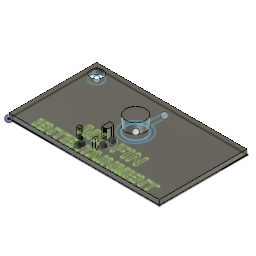
Sotto v2 (Autodesk Fusion 360 design; units mm, degrees)
Autodesk Fusion 360 part; units mm, degrees
sketch "Schizzo1" plane through (0, 0, 0) normal (0, 0, 1) x (1, 0, 0)
  line L0 (0, 0) -> (60, 0)
  line L1 (60, 0) -> (60, 35)
  line L2 (60, 35) -> (0, 35)
  line L3 (0, 35) -> (0, 0)
  circle A0 centre (4, 31) radius 2.5
  line L4 (28.9097, 26.0707) -> (28.9097, 32.0707)
  line L5 (30.9097, 32.0707) -> (30.9097, 26.0707)
  arc A1 (30.9097, 32.0707) -> (28.9097, 32.0707) centre (29.9097, 32.0707) ccw
  circle A2 centre (29.9097, 20.6624) radius 4
  line L6 (19.9916, 9.7411) -> (19.2036, 12.8732)
  line L7 (19.2036, 12.8732) -> (19.2036, 9.4795)
  spline S0 degree 2 poles (19.2036, 9.4795) (19.2036, 9.1979) (19.0778, 9.057) knots 0 0 0 1 1 1
  spline S1 degree 2 poles (19.0778, 9.057) (18.952, 8.9162) (18.7441, 8.9162) knots 0 0 0 1 1 1
  spline S2 degree 2 poles (18.7441, 8.9162) (18.5429, 8.9162) (18.4155, 9.0553) knots 0 0 0 1 1 1
  spline S3 degree 2 poles (18.4155, 9.0553) (18.2881, 9.1945) (18.2881, 9.4795) knots 0 0 0 1 1 1
  line L8 (18.2881, 9.4795) -> (18.2881, 13.3696)
  spline S4 degree 2 poles (18.2881, 13.3696) (18.2881, 13.6915) (18.4557, 13.8038) knots 0 0 0 1 1 1
  spline S5 degree 2 poles (18.4557, 13.8038) (18.6234, 13.9162) (18.9085, 13.9162) knots 0 0 0 1 1 1
  line L9 (18.9085, 13.9162) -> (19.217, 13.9162)
  spline S6 degree 2 poles (19.217, 13.9162) (19.4953, 13.9162) (19.6211, 13.8659) knots 0 0 0 1 1 1
  spline S7 degree 2 poles (19.6211, 13.8659) (19.7468, 13.8156) (19.8072, 13.6848) knots 0 0 0 1 1 1
  spline S8 degree 2 poles (19.8072, 13.6848) (19.8675, 13.554) (19.9447, 13.2589) knots 0 0 0 1 1 1
  line L10 (19.9447, 13.2589) -> (20.659, 10.5661)
  line L11 (20.659, 10.5661) -> (21.3732, 13.2589)
  spline S9 degree 2 poles (21.3732, 13.2589) (21.4504, 13.554) (21.5107, 13.6848) knots 0 0 0 1 1 1
  spline S10 degree 2 poles (21.5107, 13.6848) (21.5711, 13.8156) (21.6968, 13.8659) knots 0 0 0 1 1 1
  spline S11 degree 2 poles (21.6968, 13.8659) (21.8226, 13.9162) (22.1009, 13.9162) knots 0 0 0 1 1 1
  line L12 (22.1009, 13.9162) -> (22.4095, 13.9162)
  spline S12 degree 2 poles (22.4095, 13.9162) (22.6945, 13.9162) (22.8622, 13.8038) knots 0 0 0 1 1 1
  spline S13 degree 2 poles (22.8622, 13.8038) (23.0298, 13.6915) (23.0298, 13.3696) knots 0 0 0 1 1 1
  line L13 (23.0298, 13.3696) -> (23.0298, 9.4795)
  spline S14 degree 2 poles (23.0298, 9.4795) (23.0298, 9.1979) (22.9041, 9.057) knots 0 0 0 1 1 1
  spline S15 degree 2 poles (22.9041, 9.057) (22.7783, 8.9162) (22.5671, 8.9162) knots 0 0 0 1 1 1
  spline S16 degree 2 poles (22.5671, 8.9162) (22.3692, 8.9162) (22.2418, 9.057) knots 0 0 0 1 1 1
  spline S17 degree 2 poles (22.2418, 9.057) (22.1144, 9.1979) (22.1144, 9.4795) knots 0 0 0 1 1 1
  line L14 (22.1144, 9.4795) -> (22.1144, 12.8732)
  line L15 (22.1144, 12.8732) -> (21.3263, 9.7411)
  spline S18 degree 2 poles (21.3263, 9.7411) (21.2492, 9.4359) (21.2005, 9.2934) knots 0 0 0 1 1 1
  spline S19 degree 2 poles (21.2005, 9.2934) (21.1519, 9.1509) (21.0211, 9.0335) knots 0 0 0 1 1 1
  spline S20 degree 2 poles (21.0211, 9.0335) (20.8903, 8.9162) (20.659, 8.9162) knots 0 0 0 1 1 1
  spline S21 degree 2 poles (20.659, 8.9162) (20.4846, 8.9162) (20.3639, 8.9916) knots 0 0 0 1 1 1
  spline S22 degree 2 poles (20.3639, 8.9916) (20.2431, 9.0671) (20.1761, 9.1844) knots 0 0 0 1 1 1
  spline S23 degree 2 poles (20.1761, 9.1844) (20.109, 9.3018) (20.0704, 9.4443) knots 0 0 0 1 1 1
  spline S24 degree 2 poles (20.0704, 9.4443) (20.0319, 9.5869) (19.9916, 9.7411) knots 0 0 0 1 1 1
  line L16 (24.0929, 9.5231) -> (24.0929, 13.3964)
  spline S25 degree 2 poles (24.0929, 13.3964) (24.0929, 13.6982) (24.2304, 13.8491) knots 0 0 0 1 1 1
  spline S26 degree 2 poles (24.2304, 13.8491) (24.3679, 14) (24.5858, 14) knots 0 0 0 1 1 1
  spline S27 degree 2 poles (24.5858, 14) (24.8105, 14) (24.9497, 13.8508) knots 0 0 0 1 1 1
  spline S28 degree 2 poles (24.9497, 13.8508) (25.0889, 13.7015) (25.0889, 13.3964) knots 0 0 0 1 1 1
  line L17 (25.0889, 13.3964) -> (25.0889, 9.5231)
  spline S29 degree 2 poles (25.0889, 9.5231) (25.0889, 9.218) (24.9497, 9.0671) knots 0 0 0 1 1 1
  spline S30 degree 2 poles (24.9497, 9.0671) (24.8105, 8.9162) (24.5858, 8.9162) knots 0 0 0 1 1 1
  spline S31 degree 2 poles (24.5858, 8.9162) (24.3712, 8.9162) (24.2321, 9.0687) knots 0 0 0 1 1 1
  spline S32 degree 2 poles (24.2321, 9.0687) (24.0929, 9.2213) (24.0929, 9.5231) knots 0 0 0 1 1 1
  line L18 (26.8192, 13.9162) -> (28.117, 13.9162)
  spline S33 degree 2 poles (28.117, 13.9162) (28.6234, 13.9162) (28.9856, 13.8223) knots 0 0 0 1 1 1
  spline S34 degree 2 poles (28.9856, 13.8223) (29.3478, 13.7284) (29.6429, 13.4702) knots 0 0 0 1 1 1
  spline S35 degree 2 poles (29.6429, 13.4702) (30.4108, 12.8129) (30.4108, 11.4715) knots 0 0 0 1 1 1
  spline S36 degree 2 poles (30.4108, 11.4715) (30.4108, 11.0288) (30.3337, 10.6633) knots 0 0 0 1 1 1
  spline S37 degree 2 poles (30.3337, 10.6633) (30.2565, 10.2978) (30.0956, 10.0044) knots 0 0 0 1 1 1
  spline S38 degree 2 poles (30.0956, 10.0044) (29.9346, 9.7109) (29.6831, 9.4795) knots 0 0 0 1 1 1
  spline S39 degree 2 poles (29.6831, 9.4795) (29.4852, 9.3018) (29.2505, 9.1945) knots 0 0 0 1 1 1
  spline S40 degree 2 poles (29.2505, 9.1945) (29.0158, 9.0872) (28.7458, 9.0436) knots 0 0 0 1 1 1
  spline S41 degree 2 poles (28.7458, 9.0436) (28.4759, 9) (28.1372, 9) knots 0 0 0 1 1 1
  line L19 (28.1372, 9) -> (26.8394, 9)
  spline S42 degree 2 poles (26.8394, 9) (26.5677, 9) (26.4302, 9.0822) knots 0 0 0 1 1 1
  spline S43 degree 2 poles (26.4302, 9.0822) (26.2928, 9.1643) (26.2508, 9.3135) knots 0 0 0 1 1 1
  spline S44 degree 2 poles (26.2508, 9.3135) (26.2089, 9.4628) (26.2089, 9.7009) knots 0 0 0 1 1 1
  line L20 (26.2089, 9.7009) -> (26.2089, 13.3058)
  spline S45 degree 2 poles (26.2089, 13.3058) (26.2089, 13.6278) (26.3531, 13.772) knots 0 0 0 1 1 1
  spline S46 degree 2 poles (26.3531, 13.772) (26.4973, 13.9162) (26.8192, 13.9162) knots 0 0 0 1 1 1
  line L21 (27.2049, 13.1281) -> (27.2049, 9.7914)
  line L22 (27.2049, 9.7914) -> (27.9594, 9.7914)
  spline S47 degree 2 poles (27.9594, 9.7914) (28.2076, 9.7914) (28.3484, 9.8048) knots 0 0 0 1 1 1
  spline S48 degree 2 poles (28.3484, 9.8048) (28.4893, 9.8182) (28.6402, 9.8719) knots 0 0 0 1 1 1
  spline S49 degree 2 poles (28.6402, 9.8719) (28.7911, 9.9256) (28.9017, 10.0228) knots 0 0 0 1 1 1
  spline S50 degree 2 poles (28.9017, 10.0228) (29.4014, 10.4453) (29.4014, 11.4782) knots 0 0 0 1 1 1
  spline S51 degree 2 poles (29.4014, 11.4782) (29.4014, 12.2059) (29.1818, 12.5681) knots 0 0 0 1 1 1
  spline S52 degree 2 poles (29.1818, 12.5681) (28.9621, 12.9302) (28.6402, 13.0292) knots 0 0 0 1 1 1
  spline S53 degree 2 poles (28.6402, 13.0292) (28.3182, 13.1281) (27.8622, 13.1281) knots 0 0 0 1 1 1
  line L23 (27.8622, 13.1281) -> (27.2049, 13.1281)
  line L24 (34.2237, 13.1482) -> (32.2619, 13.1482)
  line L25 (32.2619, 13.1482) -> (32.2619, 11.8907)
  line L26 (32.2619, 11.8907) -> (33.9017, 11.8907)
  spline S54 degree 2 poles (33.9017, 11.8907) (34.1298, 11.8907) (34.2421, 11.7884) knots 0 0 0 1 1 1
  spline S55 degree 2 poles (34.2421, 11.7884) (34.3545, 11.6861) (34.3545, 11.5151) knots 0 0 0 1 1 1
  spline S56 degree 2 poles (34.3545, 11.5151) (34.3545, 11.3441) (34.2404, 11.2435) knots 0 0 0 1 1 1
  spline S57 degree 2 poles (34.2404, 11.2435) (34.1264, 11.1429) (33.9017, 11.1429) knots 0 0 0 1 1 1
  line L27 (33.9017, 11.1429) -> (32.2619, 11.1429)
  line L28 (32.2619, 11.1429) -> (32.2619, 9.5231)
  spline S58 degree 2 poles (32.2619, 9.5231) (32.2619, 9.2146) (32.1227, 9.0654) knots 0 0 0 1 1 1
  spline S59 degree 2 poles (32.1227, 9.0654) (31.9836, 8.9162) (31.7656, 8.9162) knots 0 0 0 1 1 1
  spline S60 degree 2 poles (31.7656, 8.9162) (31.5443, 8.9162) (31.4051, 9.0671) knots 0 0 0 1 1 1
  spline S61 degree 2 poles (31.4051, 9.0671) (31.2659, 9.218) (31.2659, 9.5231) knots 0 0 0 1 1 1
  line L29 (31.2659, 9.5231) -> (31.2659, 13.3058)
  spline S62 degree 2 poles (31.2659, 13.3058) (31.2659, 13.5205) (31.3296, 13.6563) knots 0 0 0 1 1 1
  spline S63 degree 2 poles (31.3296, 13.6563) (31.3934, 13.7921) (31.5292, 13.8541) knots 0 0 0 1 1 1
  spline S64 degree 2 poles (31.5292, 13.8541) (31.665, 13.9162) (31.8763, 13.9162) knots 0 0 0 1 1 1
  line L30 (31.8763, 13.9162) -> (34.2237, 13.9162)
  spline S65 degree 2 poles (34.2237, 13.9162) (34.4618, 13.9162) (34.5775, 13.8105) knots 0 0 0 1 1 1
  spline S66 degree 2 poles (34.5775, 13.8105) (34.6932, 13.7049) (34.6932, 13.5339) knots 0 0 0 1 1 1
  spline S67 degree 2 poles (34.6932, 13.5339) (34.6932, 13.3595) (34.5775, 13.2539) knots 0 0 0 1 1 1
  spline S68 degree 2 poles (34.5775, 13.2539) (34.4618, 13.1482) (34.2237, 13.1482) knots 0 0 0 1 1 1
  line L31 (35.4745, 9.5231) -> (35.4745, 13.3964)
  spline S69 degree 2 poles (35.4745, 13.3964) (35.4745, 13.6982) (35.612, 13.8491) knots 0 0 0 1 1 1
  spline S70 degree 2 poles (35.612, 13.8491) (35.7495, 14) (35.9675, 14) knots 0 0 0 1 1 1
  spline S71 degree 2 poles (35.9675, 14) (36.1922, 14) (36.3313, 13.8508) knots 0 0 0 1 1 1
  spline S72 degree 2 poles (36.3313, 13.8508) (36.4705, 13.7015) (36.4705, 13.3964) knots 0 0 0 1 1 1
  line L32 (36.4705, 13.3964) -> (36.4705, 9.5231)
  spline S73 degree 2 poles (36.4705, 9.5231) (36.4705, 9.218) (36.3313, 9.0671) knots 0 0 0 1 1 1
  spline S74 degree 2 poles (36.3313, 9.0671) (36.1922, 8.9162) (35.9675, 8.9162) knots 0 0 0 1 1 1
  spline S75 degree 2 poles (35.9675, 8.9162) (35.7529, 8.9162) (35.6137, 9.0687) knots 0 0 0 1 1 1
  spline S76 degree 2 poles (35.6137, 9.0687) (35.4745, 9.2213) (35.4745, 9.5231) knots 0 0 0 1 1 1
  line L33 (38.8816, 13.4031) -> (40.7964, 10.5057)
  line L34 (40.7964, 10.5057) -> (40.7964, 13.4299)
  spline S77 degree 2 poles (40.7964, 13.4299) (40.7964, 13.715) (40.9188, 13.8575) knots 0 0 0 1 1 1
  spline S78 degree 2 poles (40.9188, 13.8575) (41.0412, 14) (41.2492, 14) knots 0 0 0 1 1 1
  spline S79 degree 2 poles (41.2492, 14) (41.4638, 14) (41.5879, 13.8575) knots 0 0 0 1 1 1
  spline S80 degree 2 poles (41.5879, 13.8575) (41.7119, 13.715) (41.7119, 13.4299) knots 0 0 0 1 1 1
  line L35 (41.7119, 13.4299) -> (41.7119, 9.5634)
  spline S81 degree 2 poles (41.7119, 9.5634) (41.7119, 8.9162) (41.1754, 8.9162) knots 0 0 0 1 1 1
  spline S82 degree 2 poles (41.1754, 8.9162) (41.0412, 8.9162) (40.9339, 8.9547) knots 0 0 0 1 1 1
  spline S83 degree 2 poles (40.9339, 8.9547) (40.8266, 8.9933) (40.7327, 9.0771) knots 0 0 0 1 1 1
  spline S84 degree 2 poles (40.7327, 9.0771) (40.6388, 9.161) (40.5583, 9.2733) knots 0 0 0 1 1 1
  spline S85 degree 2 poles (40.5583, 9.2733) (40.4779, 9.3856) (40.3974, 9.503) knots 0 0 0 1 1 1
  line L36 (40.3974, 9.503) -> (38.5295, 12.3669)
  line L37 (38.5295, 12.3669) -> (38.5295, 9.4863)
  spline S86 degree 2 poles (38.5295, 9.4863) (38.5295, 9.2046) (38.3987, 9.0604) knots 0 0 0 1 1 1
  spline S87 degree 2 poles (38.3987, 9.0604) (38.2679, 8.9162) (38.0634, 8.9162) knots 0 0 0 1 1 1
  spline S88 degree 2 poles (38.0634, 8.9162) (37.8521, 8.9162) (37.7247, 9.062) knots 0 0 0 1 1 1
  spline S89 degree 2 poles (37.7247, 9.062) (37.5973, 9.2079) (37.5973, 9.4863) knots 0 0 0 1 1 1
  line L38 (37.5973, 9.4863) -> (37.5973, 13.279)
  spline S90 degree 2 poles (37.5973, 13.279) (37.5973, 13.5205) (37.6509, 13.6579) knots 0 0 0 1 1 1
  spline S91 degree 2 poles (37.6509, 13.6579) (37.7146, 13.8089) (37.8622, 13.9044) knots 0 0 0 1 1 1
  spline S92 degree 2 poles (37.8622, 13.9044) (38.0097, 14) (38.1808, 14) knots 0 0 0 1 1 1
  spline S93 degree 2 poles (38.1808, 14) (38.3149, 14) (38.4105, 13.9564) knots 0 0 0 1 1 1
  spline S94 degree 2 poles (38.4105, 13.9564) (38.506, 13.9128) (38.5781, 13.839) knots 0 0 0 1 1 1
  spline S95 degree 2 poles (38.5781, 13.839) (38.6502, 13.7653) (38.7257, 13.6479) knots 0 0 0 1 1 1
  spline S96 degree 2 poles (38.7257, 13.6479) (38.8011, 13.5305) (38.8816, 13.4031) knots 0 0 0 1 1 1
  line L39 (9.1089, 5.8116) -> (7.3142, 5.7974)
  line L40 (7.3142, 5.7974) -> (7.3218, 4.8316)
  line L41 (7.3218, 4.8316) -> (8.9744, 4.8447)
  spline S97 degree 2 poles (8.9744, 4.8447) (9.1568, 4.8462) (9.2473, 4.7651) knots 0 0 0 1 1 1
  spline S98 degree 2 poles (9.2473, 4.7651) (9.3378, 4.6839) (9.3389, 4.5498) knots 0 0 0 1 1 1
  spline S99 degree 2 poles (9.3389, 4.5498) (9.34, 4.4157) (9.2521, 4.3305) knots 0 0 0 1 1 1
  spline S100 degree 2 poles (9.2521, 4.3305) (9.1642, 4.2453) (8.9791, 4.2438) knots 0 0 0 1 1 1
  line L42 (8.9791, 4.2438) -> (7.3266, 4.2307)
  line L43 (7.3266, 4.2307) -> (7.3355, 3.112)
  line L44 (7.3355, 3.112) -> (9.1919, 3.1267)
  spline S101 degree 2 poles (9.1919, 3.1267) (9.3797, 3.1282) (9.4756, 3.0418) knots 0 0 0 1 1 1
  spline S102 degree 2 poles (9.4756, 3.0418) (9.5715, 2.9554) (9.5727, 2.8105) knots 0 0 0 1 1 1
  spline S103 degree 2 poles (9.5727, 2.8105) (9.5738, 2.671) (9.4793, 2.5831) knots 0 0 0 1 1 1
  spline S104 degree 2 poles (9.4793, 2.5831) (9.3847, 2.4951) (9.1969, 2.4936) knots 0 0 0 1 1 1
  line L45 (9.1969, 2.4936) -> (7.032, 2.4764)
  spline S105 degree 2 poles (7.032, 2.4764) (6.7718, 2.4744) (6.6569, 2.5888) knots 0 0 0 1 1 1
  spline S106 degree 2 poles (6.6569, 2.5888) (6.5419, 2.7033) (6.5399, 2.9608) knots 0 0 0 1 1 1
  line L46 (6.5399, 2.9608) -> (6.5164, 5.9171)
  spline S107 degree 2 poles (6.5164, 5.9171) (6.515, 6.0888) (6.5651, 6.1979) knots 0 0 0 1 1 1
  spline S108 degree 2 poles (6.5651, 6.1979) (6.6153, 6.3069) (6.7235, 6.3574) knots 0 0 0 1 1 1
  spline S109 degree 2 poles (6.7235, 6.3574) (6.8318, 6.4079) (7.0008, 6.4092) knots 0 0 0 1 1 1
  line L47 (7.0008, 6.4092) -> (9.104, 6.4259)
  spline S110 degree 2 poles (9.104, 6.4259) (9.2945, 6.4275) (9.3877, 6.3437) knots 0 0 0 1 1 1
  spline S111 degree 2 poles (9.3877, 6.3437) (9.4809, 6.2599) (9.482, 6.1231) knots 0 0 0 1 1 1
  spline S112 degree 2 poles (9.482, 6.1231) (9.4831, 5.9836) (9.3912, 5.8984) knots 0 0 0 1 1 1
  spline S113 degree 2 poles (9.3912, 5.8984) (9.2993, 5.8131) (9.1089, 5.8116) knots 0 0 0 1 1 1
  line L48 (11.2185, 6.0323) -> (12.7687, 3.7266)
  line L49 (12.7687, 3.7266) -> (12.7502, 6.0659)
  spline S114 degree 2 poles (12.7502, 6.0659) (12.7483, 6.2939) (12.8454, 6.4087) knots 0 0 0 1 1 1
  spline S115 degree 2 poles (12.8454, 6.4087) (12.9424, 6.5235) (13.1087, 6.5248) knots 0 0 0 1 1 1
  spline S116 degree 2 poles (13.1087, 6.5248) (13.2804, 6.5262) (13.3806, 6.413) knots 0 0 0 1 1 1
  spline S117 degree 2 poles (13.3806, 6.413) (13.4807, 6.2997) (13.4825, 6.0717) knots 0 0 0 1 1 1
  line L50 (13.4825, 6.0717) -> (13.5071, 2.9786)
  spline S118 degree 2 poles (13.5071, 2.9786) (13.5112, 2.4608) (13.082, 2.4574) knots 0 0 0 1 1 1
  spline S119 degree 2 poles (13.082, 2.4574) (12.9747, 2.4566) (12.8886, 2.4867) knots 0 0 0 1 1 1
  spline S120 degree 2 poles (12.8886, 2.4867) (12.8025, 2.5169) (12.7269, 2.5834) knots 0 0 0 1 1 1
  spline S121 degree 2 poles (12.7269, 2.5834) (12.6512, 2.6498) (12.5861, 2.7392) knots 0 0 0 1 1 1
  spline S122 degree 2 poles (12.5861, 2.7392) (12.521, 2.8286) (12.4559, 2.9219) knots 0 0 0 1 1 1
  line L51 (12.4559, 2.9219) -> (10.9434, 5.2011)
  line L52 (10.9434, 5.2011) -> (10.9617, 2.8967)
  spline S123 degree 2 poles (10.9617, 2.8967) (10.9635, 2.6713) (10.8598, 2.5551) knots 0 0 0 1 1 1
  spline S124 degree 2 poles (10.8598, 2.5551) (10.7561, 2.4389) (10.5925, 2.4376) knots 0 0 0 1 1 1
  spline S125 degree 2 poles (10.5925, 2.4376) (10.4235, 2.4363) (10.3206, 2.5522) knots 0 0 0 1 1 1
  spline S126 degree 2 poles (10.3206, 2.5522) (10.2177, 2.6681) (10.2159, 2.8907) knots 0 0 0 1 1 1
  line L53 (10.2159, 2.8907) -> (10.1918, 5.9248)
  spline S127 degree 2 poles (10.1918, 5.9248) (10.1903, 6.118) (10.2324, 6.2283) knots 0 0 0 1 1 1
  spline S128 degree 2 poles (10.2324, 6.2283) (10.2824, 6.3495) (10.3998, 6.4268) knots 0 0 0 1 1 1
  spline S129 degree 2 poles (10.3998, 6.4268) (10.5172, 6.5042) (10.654, 6.5053) knots 0 0 0 1 1 1
  spline S130 degree 2 poles (10.654, 6.5053) (10.7614, 6.5062) (10.8381, 6.4719) knots 0 0 0 1 1 1
  spline S131 degree 2 poles (10.8381, 6.4719) (10.9148, 6.4376) (10.973, 6.3791) knots 0 0 0 1 1 1
  spline S132 degree 2 poles (10.973, 6.3791) (11.0311, 6.3205) (11.0922, 6.2271) knots 0 0 0 1 1 1
  spline S133 degree 2 poles (11.0922, 6.2271) (11.1533, 6.1337) (11.2185, 6.0323) knots 0 0 0 1 1 1
  line L54 (16.9104, 5.8307) -> (16.0413, 5.8238)
  line L55 (16.0413, 5.8238) -> (16.064, 2.9667)
  spline S134 degree 2 poles (16.064, 2.9667) (16.0659, 2.7199) (15.9569, 2.5996) knots 0 0 0 1 1 1
  spline S135 degree 2 poles (15.9569, 2.5996) (15.8478, 2.4794) (15.6735, 2.478) knots 0 0 0 1 1 1
  spline S136 degree 2 poles (15.6735, 2.478) (15.4964, 2.4766) (15.3841, 2.5964) knots 0 0 0 1 1 1
  spline S137 degree 2 poles (15.3841, 2.5964) (15.2718, 2.7163) (15.2699, 2.9604) knots 0 0 0 1 1 1
  line L56 (15.2699, 2.9604) -> (15.2472, 5.8174)
  line L57 (15.2472, 5.8174) -> (14.378, 5.8105)
  spline S138 degree 2 poles (14.378, 5.8105) (14.1741, 5.8089) (14.0741, 5.898) knots 0 0 0 1 1 1
  spline S139 degree 2 poles (14.0741, 5.898) (13.9742, 5.9871) (13.973, 6.1346) knots 0 0 0 1 1 1
  spline S140 degree 2 poles (13.973, 6.1346) (13.9718, 6.2875) (14.0744, 6.3769) knots 0 0 0 1 1 1
  spline S141 degree 2 poles (14.0744, 6.3769) (14.1769, 6.4662) (14.3728, 6.4678) knots 0 0 0 1 1 1
  line L58 (14.3728, 6.4678) -> (16.9052, 6.4879)
  spline S142 degree 2 poles (16.9052, 6.4879) (17.1118, 6.4896) (17.2131, 6.3991) knots 0 0 0 1 1 1
  spline S143 degree 2 poles (17.2131, 6.3991) (17.3144, 6.3087) (17.3156, 6.1612) knots 0 0 0 1 1 1
  spline S144 degree 2 poles (17.3156, 6.1612) (17.3168, 6.0136) (17.2156, 5.923) knots 0 0 0 1 1 1
  spline S145 degree 2 poles (17.2156, 5.923) (17.1143, 5.8323) (16.9104, 5.8307) knots 0 0 0 1 1 1
  line L59 (20.3815, 5.9012) -> (18.5868, 5.8869)
  line L60 (18.5868, 5.8869) -> (18.5944, 4.9211)
  line L61 (18.5944, 4.9211) -> (20.247, 4.9343)
  spline S146 degree 2 poles (20.247, 4.9343) (20.4294, 4.9357) (20.5199, 4.8546) knots 0 0 0 1 1 1
  spline S147 degree 2 poles (20.5199, 4.8546) (20.6104, 4.7735) (20.6115, 4.6394) knots 0 0 0 1 1 1
  spline S148 degree 2 poles (20.6115, 4.6394) (20.6126, 4.5052) (20.5247, 4.42) knots 0 0 0 1 1 1
  spline S149 degree 2 poles (20.5247, 4.42) (20.4369, 4.3348) (20.2517, 4.3333) knots 0 0 0 1 1 1
  line L62 (20.2517, 4.3333) -> (18.5992, 4.3202)
  line L63 (18.5992, 4.3202) -> (18.6081, 3.2015)
  line L64 (18.6081, 3.2015) -> (20.4645, 3.2163)
  spline S150 degree 2 poles (20.4645, 3.2163) (20.6523, 3.2178) (20.7482, 3.1313) knots 0 0 0 1 1 1
  spline S151 degree 2 poles (20.7482, 3.1313) (20.8442, 3.0449) (20.8453, 2.9001) knots 0 0 0 1 1 1
  spline S152 degree 2 poles (20.8453, 2.9001) (20.8464, 2.7606) (20.7519, 2.6726) knots 0 0 0 1 1 1
  spline S153 degree 2 poles (20.7519, 2.6726) (20.6573, 2.5847) (20.4695, 2.5832) knots 0 0 0 1 1 1
  line L65 (20.4695, 2.5832) -> (18.3046, 2.566)
  spline S154 degree 2 poles (18.3046, 2.566) (18.0444, 2.5639) (17.9295, 2.6784) knots 0 0 0 1 1 1
  spline S155 degree 2 poles (17.9295, 2.6784) (17.8145, 2.7928) (17.8125, 3.0503) knots 0 0 0 1 1 1
  line L66 (17.8125, 3.0503) -> (17.789, 6.0067)
  spline S156 degree 2 poles (17.789, 6.0067) (17.7877, 6.1783) (17.8378, 6.2874) knots 0 0 0 1 1 1
  spline S157 degree 2 poles (17.8378, 6.2874) (17.8879, 6.3965) (17.9961, 6.4469) knots 0 0 0 1 1 1
  spline S158 degree 2 poles (17.9961, 6.4469) (18.1044, 6.4974) (18.2734, 6.4988) knots 0 0 0 1 1 1
  line L67 (18.2734, 6.4988) -> (20.3766, 6.5155)
  spline S159 degree 2 poles (20.3766, 6.5155) (20.5671, 6.517) (20.6603, 6.4332) knots 0 0 0 1 1 1
  spline S160 degree 2 poles (20.6603, 6.4332) (20.7535, 6.3495) (20.7546, 6.2126) knots 0 0 0 1 1 1
  spline S161 degree 2 poles (20.7546, 6.2126) (20.7557, 6.0731) (20.6638, 5.9879) knots 0 0 0 1 1 1
  spline S162 degree 2 poles (20.6638, 5.9879) (20.572, 5.9027) (20.3815, 5.9012) knots 0 0 0 1 1 1
  line L68 (22.5379, 4.2817) -> (22.2589, 4.2795)
  line L69 (22.2589, 4.2795) -> (22.269, 3.016)
  spline S163 degree 2 poles (22.269, 3.016) (22.271, 2.7665) (22.1619, 2.6476) knots 0 0 0 1 1 1
  spline S164 degree 2 poles (22.1619, 2.6476) (22.0529, 2.5287) (21.8758, 2.5273) knots 0 0 0 1 1 1
  spline S165 degree 2 poles (21.8758, 2.5273) (21.6853, 2.5258) (21.5797, 2.6483) knots 0 0 0 1 1 1
  spline S166 degree 2 poles (21.5797, 2.6483) (21.4741, 2.7709) (21.4722, 3.0097) knots 0 0 0 1 1 1
  line L70 (21.4722, 3.0097) -> (21.4482, 6.0357)
  spline S167 degree 2 poles (21.4482, 6.0357) (21.4461, 6.2933) (21.5606, 6.4095) knots 0 0 0 1 1 1
  spline S168 degree 2 poles (21.5606, 6.4095) (21.675, 6.5258) (21.9326, 6.5278) knots 0 0 0 1 1 1
  line L71 (21.9326, 6.5278) -> (23.2283, 6.5381)
  spline S169 degree 2 poles (23.2283, 6.5381) (23.4966, 6.5403) (23.6872, 6.519) knots 0 0 0 1 1 1
  spline S170 degree 2 poles (23.6872, 6.519) (23.8779, 6.4977) (24.0313, 6.4292) knots 0 0 0 1 1 1
  spline S171 degree 2 poles (24.0313, 6.4292) (24.2171, 6.3528) (24.3604, 6.2091) knots 0 0 0 1 1 1
  spline S172 degree 2 poles (24.3604, 6.2091) (24.5037, 6.0654) (24.579, 5.8741) knots 0 0 0 1 1 1
  spline S173 degree 2 poles (24.579, 5.8741) (24.6543, 5.6829) (24.656, 5.4683) knots 0 0 0 1 1 1
  spline S174 degree 2 poles (24.656, 5.4683) (24.6595, 5.0283) (24.4135, 4.7635) knots 0 0 0 1 1 1
  spline S175 degree 2 poles (24.4135, 4.7635) (24.1674, 4.4986) (23.6639, 4.3846) knots 0 0 0 1 1 1
  spline S176 degree 2 poles (23.6639, 4.3846) (23.8768, 4.2736) (24.0717, 4.0552) knots 0 0 0 1 1 1
  spline S177 degree 2 poles (24.0717, 4.0552) (24.2666, 3.8367) (24.4201, 3.5898) knots 0 0 0 1 1 1
  spline S178 degree 2 poles (24.4201, 3.5898) (24.5736, 3.3428) (24.6597, 3.1436) knots 0 0 0 1 1 1
  spline S179 degree 2 poles (24.6597, 3.1436) (24.7458, 2.9445) (24.7464, 2.8693) knots 0 0 0 1 1 1
  spline S180 degree 2 poles (24.7464, 2.8693) (24.747, 2.7915) (24.698, 2.7147) knots 0 0 0 1 1 1
  spline S181 degree 2 poles (24.698, 2.7147) (24.649, 2.6378) (24.5635, 2.5929) knots 0 0 0 1 1 1
  spline S182 degree 2 poles (24.5635, 2.5929) (24.478, 2.5479) (24.3653, 2.547) knots 0 0 0 1 1 1
  spline S183 degree 2 poles (24.3653, 2.547) (24.2312, 2.546) (24.1395, 2.6083) knots 0 0 0 1 1 1
  spline S184 degree 2 poles (24.1395, 2.6083) (24.0478, 2.6706) (23.9813, 2.7667) knots 0 0 0 1 1 1
  spline S185 degree 2 poles (23.9813, 2.7667) (23.9148, 2.8627) (23.8006, 3.0496) knots 0 0 0 1 1 1
  line L72 (23.8006, 3.0496) -> (23.4772, 3.5783)
  spline S186 degree 2 poles (23.4772, 3.5783) (23.3032, 3.8693) (23.1665, 4.0211) knots 0 0 0 1 1 1
  spline S187 degree 2 poles (23.1665, 4.0211) (23.0298, 4.173) (22.8898, 4.2282) knots 0 0 0 1 1 1
  spline S188 degree 2 poles (22.8898, 4.2282) (22.7499, 4.2834) (22.5379, 4.2817) knots 0 0 0 1 1 1
  line L73 (22.9809, 5.9379) -> (22.2458, 5.9321)
  line L74 (22.2458, 5.9321) -> (22.2544, 4.8509)
  line L75 (22.2544, 4.8509) -> (22.968, 4.8566)
  spline S189 degree 2 poles (22.968, 4.8566) (23.255, 4.8589) (23.4505, 4.9101) knots 0 0 0 1 1 1
  spline S190 degree 2 poles (23.4505, 4.9101) (23.6459, 4.9613) (23.7483, 5.0815) knots 0 0 0 1 1 1
  spline S191 degree 2 poles (23.7483, 5.0815) (23.8506, 5.2017) (23.8489, 5.4109) knots 0 0 0 1 1 1
  spline S192 degree 2 poles (23.8489, 5.4109) (23.8476, 5.5746) (23.7635, 5.6986) knots 0 0 0 1 1 1
  spline S193 degree 2 poles (23.7635, 5.6986) (23.6793, 5.8227) (23.5313, 5.8833) knots 0 0 0 1 1 1
  spline S194 degree 2 poles (23.5313, 5.8833) (23.3913, 5.9412) (22.9809, 5.9379) knots 0 0 0 1 1 1
  line L76 (27.6868, 5.9163) -> (26.8176, 5.9094)
  line L77 (26.8176, 5.9094) -> (26.8403, 3.0523)
  spline S195 degree 2 poles (26.8403, 3.0523) (26.8422, 2.8055) (26.7332, 2.6852) knots 0 0 0 1 1 1
  spline S196 degree 2 poles (26.7332, 2.6852) (26.6241, 2.565) (26.4498, 2.5636) knots 0 0 0 1 1 1
  spline S197 degree 2 poles (26.4498, 2.5636) (26.2727, 2.5622) (26.1604, 2.682) knots 0 0 0 1 1 1
  spline S198 degree 2 poles (26.1604, 2.682) (26.0481, 2.8019) (26.0462, 3.046) knots 0 0 0 1 1 1
  line L78 (26.0462, 3.046) -> (26.0235, 5.903)
  line L79 (26.0235, 5.903) -> (25.1543, 5.8961)
  spline S199 degree 2 poles (25.1543, 5.8961) (24.9504, 5.8945) (24.8505, 5.9836) knots 0 0 0 1 1 1
  spline S200 degree 2 poles (24.8505, 5.9836) (24.7505, 6.0727) (24.7493, 6.2202) knots 0 0 0 1 1 1
  spline S201 degree 2 poles (24.7493, 6.2202) (24.7481, 6.3731) (24.8507, 6.4625) knots 0 0 0 1 1 1
  spline S202 degree 2 poles (24.8507, 6.4625) (24.9533, 6.5518) (25.1491, 6.5534) knots 0 0 0 1 1 1
  line L80 (25.1491, 6.5534) -> (27.6815, 6.5735)
  spline S203 degree 2 poles (27.6815, 6.5735) (27.8881, 6.5752) (27.9894, 6.4847) knots 0 0 0 1 1 1
  spline S204 degree 2 poles (27.9894, 6.4847) (28.0908, 6.3943) (28.0919, 6.2468) knots 0 0 0 1 1 1
  spline S205 degree 2 poles (28.0919, 6.2468) (28.0931, 6.0992) (27.9919, 6.0086) knots 0 0 0 1 1 1
  spline S206 degree 2 poles (27.9919, 6.0086) (27.8906, 5.9179) (27.6868, 5.9163) knots 0 0 0 1 1 1
  line L81 (30.7594, 3.1103) -> (30.5677, 3.6024)
  line L82 (30.5677, 3.6024) -> (28.9689, 3.5897)
  line L83 (28.9689, 3.5897) -> (28.7851, 3.0839)
  spline S207 degree 2 poles (28.7851, 3.0839) (28.6774, 2.7879) (28.6005, 2.684) knots 0 0 0 1 1 1
  spline S208 degree 2 poles (28.6005, 2.684) (28.5235, 2.5801) (28.3464, 2.5787) knots 0 0 0 1 1 1
  spline S209 degree 2 poles (28.3464, 2.5787) (28.1962, 2.5775) (28.08, 2.6866) knots 0 0 0 1 1 1
  spline S210 degree 2 poles (28.08, 2.6866) (27.9637, 2.7956) (27.9626, 2.9351) knots 0 0 0 1 1 1
  spline S211 degree 2 poles (27.9626, 2.9351) (27.962, 3.0156) (27.9881, 3.1017) knots 0 0 0 1 1 1
  spline S212 degree 2 poles (27.9881, 3.1017) (28.0143, 3.1877) (28.0748, 3.3411) knots 0 0 0 1 1 1
  line L84 (28.0748, 3.3411) -> (29.0605, 5.903)
  spline S213 degree 2 poles (29.0605, 5.903) (29.1025, 6.0134) (29.1617, 6.1681) knots 0 0 0 1 1 1
  spline S214 degree 2 poles (29.1617, 6.1681) (29.2208, 6.3228) (29.2884, 6.4253) knots 0 0 0 1 1 1
  spline S215 degree 2 poles (29.2884, 6.4253) (29.356, 6.5278) (29.4668, 6.5917) knots 0 0 0 1 1 1
  spline S216 degree 2 poles (29.4668, 6.5917) (29.5777, 6.6557) (29.7413, 6.657) knots 0 0 0 1 1 1
  spline S217 degree 2 poles (29.7413, 6.657) (29.9076, 6.6583) (30.0195, 6.5961) knots 0 0 0 1 1 1
  spline S218 degree 2 poles (30.0195, 6.5961) (30.1313, 6.534) (30.2005, 6.4352) knots 0 0 0 1 1 1
  spline S219 degree 2 poles (30.2005, 6.4352) (30.2697, 6.3365) (30.3175, 6.2229) knots 0 0 0 1 1 1
  spline S220 degree 2 poles (30.3175, 6.2229) (30.3654, 6.1092) (30.4393, 5.9193) knots 0 0 0 1 1 1
  line L85 (30.4393, 5.9193) -> (31.487, 3.3897)
  spline S221 degree 2 poles (31.487, 3.3897) (31.61, 3.1009) (31.611, 2.9695) knots 0 0 0 1 1 1
  spline S222 degree 2 poles (31.611, 2.9695) (31.6121, 2.8327) (31.499, 2.7177) knots 0 0 0 1 1 1
  spline S223 degree 2 poles (31.499, 2.7177) (31.3859, 2.6028) (31.2249, 2.6015) knots 0 0 0 1 1 1
  spline S224 degree 2 poles (31.2249, 2.6015) (31.131, 2.6008) (31.0637, 2.6338) knots 0 0 0 1 1 1
  spline S225 degree 2 poles (31.0637, 2.6338) (30.9964, 2.6668) (30.9503, 2.7241) knots 0 0 0 1 1 1
  spline S226 degree 2 poles (30.9503, 2.7241) (30.9043, 2.7814) (30.851, 2.9004) knots 0 0 0 1 1 1
  spline S227 degree 2 poles (30.851, 2.9004) (30.7977, 3.0194) (30.7594, 3.1103) knots 0 0 0 1 1 1
  line L86 (29.1734, 4.1896) -> (30.3484, 4.1989)
  line L87 (30.3484, 4.1989) -> (29.7426, 5.8172)
  line L88 (29.7426, 5.8172) -> (29.1734, 4.1896)
  line L89 (32.2271, 3.0951) -> (32.2025, 6.1936)
  spline S228 degree 2 poles (32.2025, 6.1936) (32.2006, 6.435) (32.3096, 6.5566) knots 0 0 0 1 1 1
  spline S229 degree 2 poles (32.3096, 6.5566) (32.4186, 6.6782) (32.593, 6.6796) knots 0 0 0 1 1 1
  spline S230 degree 2 poles (32.593, 6.6796) (32.7727, 6.681) (32.885, 6.5625) knots 0 0 0 1 1 1
  spline S231 degree 2 poles (32.885, 6.5625) (32.9973, 6.444) (32.9992, 6.1999) knots 0 0 0 1 1 1
  line L90 (32.9992, 6.1999) -> (33.0238, 3.1014)
  spline S232 degree 2 poles (33.0238, 3.1014) (33.0258, 2.8573) (32.9154, 2.7357) knots 0 0 0 1 1 1
  spline S233 degree 2 poles (32.9154, 2.7357) (32.805, 2.6141) (32.6253, 2.6127) knots 0 0 0 1 1 1
  spline S234 degree 2 poles (32.6253, 2.6127) (32.4536, 2.6113) (32.3413, 2.7325) knots 0 0 0 1 1 1
  spline S235 degree 2 poles (32.3413, 2.7325) (32.229, 2.8537) (32.2271, 3.0951) knots 0 0 0 1 1 1
  line L91 (34.928, 6.2206) -> (36.4783, 3.9149)
  line L92 (36.4783, 3.9149) -> (36.4597, 6.2542)
  spline S236 degree 2 poles (36.4597, 6.2542) (36.4579, 6.4823) (36.5549, 6.5971) knots 0 0 0 1 1 1
  spline S237 degree 2 poles (36.5549, 6.5971) (36.6519, 6.7118) (36.8182, 6.7132) knots 0 0 0 1 1 1
  spline S238 degree 2 poles (36.8182, 6.7132) (36.9899, 6.7145) (37.0901, 6.6013) knots 0 0 0 1 1 1
  spline S239 degree 2 poles (37.0901, 6.6013) (37.1902, 6.4881) (37.192, 6.2601) knots 0 0 0 1 1 1
  line L93 (37.192, 6.2601) -> (37.2166, 3.1669)
  spline S240 degree 2 poles (37.2166, 3.1669) (37.2207, 2.6492) (36.7915, 2.6458) knots 0 0 0 1 1 1
  spline S241 degree 2 poles (36.7915, 2.6458) (36.6842, 2.6449) (36.5981, 2.6751) knots 0 0 0 1 1 1
  spline S242 degree 2 poles (36.5981, 2.6751) (36.512, 2.7052) (36.4364, 2.7717) knots 0 0 0 1 1 1
  spline S243 degree 2 poles (36.4364, 2.7717) (36.3607, 2.8382) (36.2956, 2.9275) knots 0 0 0 1 1 1
  spline S244 degree 2 poles (36.2956, 2.9275) (36.2305, 3.0169) (36.1654, 3.1103) knots 0 0 0 1 1 1
  line L94 (36.1654, 3.1103) -> (34.6529, 5.3894)
  line L95 (34.6529, 5.3894) -> (34.6712, 3.085)
  spline S245 degree 2 poles (34.6712, 3.085) (34.673, 2.8597) (34.5693, 2.7435) knots 0 0 0 1 1 1
  spline S246 degree 2 poles (34.5693, 2.7435) (34.4656, 2.6273) (34.302, 2.626) knots 0 0 0 1 1 1
  spline S247 degree 2 poles (34.302, 2.626) (34.133, 2.6246) (34.0301, 2.7405) knots 0 0 0 1 1 1
  spline S248 degree 2 poles (34.0301, 2.7405) (33.9272, 2.8564) (33.9255, 3.0791) knots 0 0 0 1 1 1
  line L96 (33.9255, 3.0791) -> (33.9014, 6.1132)
  spline S249 degree 2 poles (33.9014, 6.1132) (33.8998, 6.3063) (33.9419, 6.4167) knots 0 0 0 1 1 1
  spline S250 degree 2 poles (33.9419, 6.4167) (33.9919, 6.5378) (34.1093, 6.6152) knots 0 0 0 1 1 1
  spline S251 degree 2 poles (34.1093, 6.6152) (34.2267, 6.6926) (34.3636, 6.6937) knots 0 0 0 1 1 1
  spline S252 degree 2 poles (34.3636, 6.6937) (34.4709, 6.6945) (34.5476, 6.6603) knots 0 0 0 1 1 1
  spline S253 degree 2 poles (34.5476, 6.6603) (34.6243, 6.626) (34.6825, 6.5674) knots 0 0 0 1 1 1
  spline S254 degree 2 poles (34.6825, 6.5674) (34.7406, 6.5089) (34.8017, 6.4155) knots 0 0 0 1 1 1
  spline S255 degree 2 poles (34.8017, 6.4155) (34.8628, 6.322) (34.928, 6.2206) knots 0 0 0 1 1 1
  line L97 (39.4153, 3.3266) -> (38.7649, 5.8272)
  line L98 (38.7649, 5.8272) -> (38.7865, 3.1123)
  spline S256 degree 2 poles (38.7865, 3.1123) (38.7883, 2.887) (38.6886, 2.7735) knots 0 0 0 1 1 1
  spline S257 degree 2 poles (38.6886, 2.7735) (38.5889, 2.66) (38.4226, 2.6587) knots 0 0 0 1 1 1
  spline S258 degree 2 poles (38.4226, 2.6587) (38.2616, 2.6574) (38.1588, 2.768) knots 0 0 0 1 1 1
  spline S259 degree 2 poles (38.1588, 2.768) (38.056, 2.8785) (38.0541, 3.1065) knots 0 0 0 1 1 1
  line L99 (38.0541, 3.1065) -> (38.0294, 6.2184)
  spline S260 degree 2 poles (38.0294, 6.2184) (38.0274, 6.476) (38.1608, 6.5669) knots 0 0 0 1 1 1
  spline S261 degree 2 poles (38.1608, 6.5669) (38.2942, 6.6578) (38.5222, 6.6596) knots 0 0 0 1 1 1
  line L100 (38.5222, 6.6596) -> (38.769, 6.6616)
  spline S262 degree 2 poles (38.769, 6.6616) (38.9917, 6.6634) (39.0926, 6.6239) knots 0 0 0 1 1 1
  spline S263 degree 2 poles (39.0926, 6.6239) (39.1936, 6.5845) (39.2427, 6.4802) knots 0 0 0 1 1 1
  spline S264 degree 2 poles (39.2427, 6.4802) (39.2918, 6.376) (39.3554, 6.1404) knots 0 0 0 1 1 1
  line L101 (39.3554, 6.1404) -> (39.9439, 3.9908)
  line L102 (39.9439, 3.9908) -> (40.4982, 6.1495)
  spline S265 degree 2 poles (40.4982, 6.1495) (40.558, 6.3861) (40.6055, 6.4911) knots 0 0 0 1 1 1
  spline S266 degree 2 poles (40.6055, 6.4911) (40.6529, 6.5961) (40.7532, 6.6371) knots 0 0 0 1 1 1
  spline S267 degree 2 poles (40.7532, 6.6371) (40.8535, 6.6782) (41.0762, 6.6799) knots 0 0 0 1 1 1
  line L103 (41.0762, 6.6799) -> (41.323, 6.6819)
  spline S268 degree 2 poles (41.323, 6.6819) (41.551, 6.6837) (41.6858, 6.5949) knots 0 0 0 1 1 1
  spline S269 degree 2 poles (41.6858, 6.5949) (41.8207, 6.5061) (41.8227, 6.2485) knots 0 0 0 1 1 1
  line L104 (41.8227, 6.2485) -> (41.8475, 3.1366)
  spline S270 degree 2 poles (41.8475, 3.1366) (41.8492, 2.9113) (41.7495, 2.7978) knots 0 0 0 1 1 1
  spline S271 degree 2 poles (41.7495, 2.7978) (41.6498, 2.6844) (41.4808, 2.683) knots 0 0 0 1 1 1
  spline S272 degree 2 poles (41.4808, 2.683) (41.3225, 2.6818) (41.2197, 2.7936) knots 0 0 0 1 1 1
  spline S273 degree 2 poles (41.2197, 2.7936) (41.1169, 2.9055) (41.1151, 3.1308) knots 0 0 0 1 1 1
  line L105 (41.1151, 3.1308) -> (41.0935, 5.8457)
  line L106 (41.0935, 5.8457) -> (40.483, 3.3351)
  spline S274 degree 2 poles (40.483, 3.3351) (40.4232, 3.0905) (40.3852, 2.9761) knots 0 0 0 1 1 1
  spline S275 degree 2 poles (40.3852, 2.9761) (40.3472, 2.8618) (40.2434, 2.7671) knots 0 0 0 1 1 1
  spline S276 degree 2 poles (40.2434, 2.7671) (40.1395, 2.6724) (39.9544, 2.6709) knots 0 0 0 1 1 1
  spline S277 degree 2 poles (39.9544, 2.6709) (39.8149, 2.6698) (39.7178, 2.7294) knots 0 0 0 1 1 1
  spline S278 degree 2 poles (39.7178, 2.7294) (39.6208, 2.789) (39.5664, 2.8824) knots 0 0 0 1 1 1
  spline S279 degree 2 poles (39.5664, 2.8824) (39.512, 2.9759) (39.4802, 3.0897) knots 0 0 0 1 1 1
  spline S280 degree 2 poles (39.4802, 3.0897) (39.4485, 3.2034) (39.4153, 3.3266) knots 0 0 0 1 1 1
  line L107 (45.2338, 6.0986) -> (43.4391, 6.0843)
  line L108 (43.4391, 6.0843) -> (43.4468, 5.1186)
  line L109 (43.4468, 5.1186) -> (45.0993, 5.1317)
  spline S281 degree 2 poles (45.0993, 5.1317) (45.2817, 5.1331) (45.3723, 5.052) knots 0 0 0 1 1 1
  spline S282 degree 2 poles (45.3723, 5.052) (45.4628, 4.9709) (45.4638, 4.8368) knots 0 0 0 1 1 1
  spline S283 degree 2 poles (45.4638, 4.8368) (45.4649, 4.7027) (45.377, 4.6174) knots 0 0 0 1 1 1
  spline S284 degree 2 poles (45.377, 4.6174) (45.2892, 4.5322) (45.1041, 4.5308) knots 0 0 0 1 1 1
  line L110 (45.1041, 4.5308) -> (43.4516, 4.5176)
  line L111 (43.4516, 4.5176) -> (43.4604, 3.399)
  line L112 (43.4604, 3.399) -> (45.3169, 3.4137)
  spline S285 degree 2 poles (45.3169, 3.4137) (45.5046, 3.4152) (45.6006, 3.3288) knots 0 0 0 1 1 1
  spline S286 degree 2 poles (45.6006, 3.3288) (45.6965, 3.2423) (45.6976, 3.0975) knots 0 0 0 1 1 1
  spline S287 degree 2 poles (45.6976, 3.0975) (45.6988, 2.958) (45.6042, 2.87) knots 0 0 0 1 1 1
  spline S288 degree 2 poles (45.6042, 2.87) (45.5097, 2.7821) (45.3219, 2.7806) knots 0 0 0 1 1 1
  line L113 (45.3219, 2.7806) -> (43.157, 2.7634)
  spline S289 degree 2 poles (43.157, 2.7634) (42.8967, 2.7613) (42.7818, 2.8758) knots 0 0 0 1 1 1
  spline S290 degree 2 poles (42.7818, 2.8758) (42.6669, 2.9902) (42.6648, 3.2478) knots 0 0 0 1 1 1
  line L114 (42.6648, 3.2478) -> (42.6414, 6.2041)
  spline S291 degree 2 poles (42.6414, 6.2041) (42.64, 6.3758) (42.6901, 6.4848) knots 0 0 0 1 1 1
  spline S292 degree 2 poles (42.6901, 6.4848) (42.7402, 6.5939) (42.8485, 6.6444) knots 0 0 0 1 1 1
  spline S293 degree 2 poles (42.8485, 6.6444) (42.9567, 6.6949) (43.1257, 6.6962) knots 0 0 0 1 1 1
  line L115 (43.1257, 6.6962) -> (45.2289, 6.7129)
  spline S294 degree 2 poles (45.2289, 6.7129) (45.4194, 6.7144) (45.5126, 6.6307) knots 0 0 0 1 1 1
  spline S295 degree 2 poles (45.5126, 6.6307) (45.6059, 6.5469) (45.6069, 6.4101) knots 0 0 0 1 1 1
  spline S296 degree 2 poles (45.6069, 6.4101) (45.6081, 6.2706) (45.5162, 6.1853) knots 0 0 0 1 1 1
  spline S297 degree 2 poles (45.5162, 6.1853) (45.4243, 6.1001) (45.2338, 6.0986) knots 0 0 0 1 1 1
  line L116 (47.3435, 6.3192) -> (48.8937, 4.0136)
  line L117 (48.8937, 4.0136) -> (48.8751, 6.3529)
  spline S298 degree 2 poles (48.8751, 6.3529) (48.8733, 6.5809) (48.9703, 6.6957) knots 0 0 0 1 1 1
  spline S299 degree 2 poles (48.9703, 6.6957) (49.0673, 6.8105) (49.2336, 6.8118) knots 0 0 0 1 1 1
  spline S300 degree 2 poles (49.2336, 6.8118) (49.4053, 6.8132) (49.5055, 6.6999) knots 0 0 0 1 1 1
  spline S301 degree 2 poles (49.5055, 6.6999) (49.6057, 6.5867) (49.6075, 6.3587) knots 0 0 0 1 1 1
  line L118 (49.6075, 6.3587) -> (49.632, 3.2656)
  spline S302 degree 2 poles (49.632, 3.2656) (49.6362, 2.7478) (49.2069, 2.7444) knots 0 0 0 1 1 1
  spline S303 degree 2 poles (49.2069, 2.7444) (49.0996, 2.7435) (49.0135, 2.7737) knots 0 0 0 1 1 1
  spline S304 degree 2 poles (49.0135, 2.7737) (48.9274, 2.8039) (48.8518, 2.8703) knots 0 0 0 1 1 1
  spline S305 degree 2 poles (48.8518, 2.8703) (48.7762, 2.9368) (48.7111, 3.0262) knots 0 0 0 1 1 1
  spline S306 degree 2 poles (48.7111, 3.0262) (48.646, 3.1155) (48.5808, 3.2089) knots 0 0 0 1 1 1
  line L119 (48.5808, 3.2089) -> (47.0684, 5.488)
  line L120 (47.0684, 5.488) -> (47.0867, 3.1836)
  spline S307 degree 2 poles (47.0867, 3.1836) (47.0885, 2.9583) (46.9848, 2.8421) knots 0 0 0 1 1 1
  spline S308 degree 2 poles (46.9848, 2.8421) (46.8811, 2.7259) (46.7174, 2.7246) knots 0 0 0 1 1 1
  spline S309 degree 2 poles (46.7174, 2.7246) (46.5484, 2.7233) (46.4455, 2.8392) knots 0 0 0 1 1 1
  spline S310 degree 2 poles (46.4455, 2.8392) (46.3427, 2.955) (46.3409, 3.1777) knots 0 0 0 1 1 1
  line L121 (46.3409, 3.1777) -> (46.3168, 6.2118)
  spline S311 degree 2 poles (46.3168, 6.2118) (46.3153, 6.405) (46.3573, 6.5153) knots 0 0 0 1 1 1
  spline S312 degree 2 poles (46.3573, 6.5153) (46.4073, 6.6364) (46.5248, 6.7138) knots 0 0 0 1 1 1
  spline S313 degree 2 poles (46.5248, 6.7138) (46.6422, 6.7912) (46.779, 6.7923) knots 0 0 0 1 1 1
  spline S314 degree 2 poles (46.779, 6.7923) (46.8863, 6.7931) (46.963, 6.7589) knots 0 0 0 1 1 1
  spline S315 degree 2 poles (46.963, 6.7589) (47.0398, 6.7246) (47.0979, 6.6661) knots 0 0 0 1 1 1
  spline S316 degree 2 poles (47.0979, 6.6661) (47.1561, 6.6075) (47.2172, 6.5141) knots 0 0 0 1 1 1
  spline S317 degree 2 poles (47.2172, 6.5141) (47.2783, 6.4207) (47.3435, 6.3192) knots 0 0 0 1 1 1
  line L122 (53.0354, 6.1176) -> (52.1662, 6.1107)
  line L123 (52.1662, 6.1107) -> (52.1889, 3.2537)
  spline S318 degree 2 poles (52.1889, 3.2537) (52.1909, 3.0069) (52.0818, 2.8866) knots 0 0 0 1 1 1
  spline S319 degree 2 poles (52.0818, 2.8866) (51.9728, 2.7664) (51.7984, 2.765) knots 0 0 0 1 1 1
  spline S320 degree 2 poles (51.7984, 2.765) (51.6213, 2.7636) (51.5091, 2.8834) knots 0 0 0 1 1 1
  spline S321 degree 2 poles (51.5091, 2.8834) (51.3968, 3.0032) (51.3948, 3.2474) knots 0 0 0 1 1 1
  line L124 (51.3948, 3.2474) -> (51.3721, 6.1044)
  line L125 (51.3721, 6.1044) -> (50.5029, 6.0975)
  spline S322 degree 2 poles (50.5029, 6.0975) (50.2991, 6.0959) (50.1991, 6.185) knots 0 0 0 1 1 1
  spline S323 degree 2 poles (50.1991, 6.185) (50.0991, 6.2741) (50.0979, 6.4216) knots 0 0 0 1 1 1
  spline S324 degree 2 poles (50.0979, 6.4216) (50.0967, 6.5745) (50.1993, 6.6639) knots 0 0 0 1 1 1
  spline S325 degree 2 poles (50.1993, 6.6639) (50.3019, 6.7532) (50.4977, 6.7548) knots 0 0 0 1 1 1
  line L126 (50.4977, 6.7548) -> (53.0302, 6.7749)
  spline S326 degree 2 poles (53.0302, 6.7749) (53.2367, 6.7765) (53.3381, 6.6861) knots 0 0 0 1 1 1
  spline S327 degree 2 poles (53.3381, 6.6861) (53.4394, 6.5957) (53.4406, 6.4482) knots 0 0 0 1 1 1
  spline S328 degree 2 poles (53.4406, 6.4482) (53.4417, 6.3006) (53.3405, 6.2099) knots 0 0 0 1 1 1
  spline S329 degree 2 poles (53.3405, 6.2099) (53.2393, 6.1192) (53.0354, 6.1176) knots 0 0 0 1 1 1
  arc A3 (28.9097, 26.0707) -> (30.9097, 26.0707) centre (29.9097, 20.6624) ccw
  spline S330 degree 3 poles (28.6989, 13.2204) (28.459, 13.2941) (28.1807, 13.3281) (27.8622, 13.3281) knots 0 0 0 0 1 1 1 1
  line L127 (27.8622, 13.3281) -> (27.0049, 13.3281)
  line L128 (27.0049, 13.3281) -> (27.0049, 9.5914)
  line L129 (27.0049, 9.5914) -> (27.9594, 9.5914)
  spline S331 degree 3 poles (27.9594, 9.5914) (28.1285, 9.5914) (28.2625, 9.5957) (28.3674, 9.6057) knots 0 0 0 0 1 1 1 1
  spline S332 degree 3 poles (28.3674, 9.6057) (28.4796, 9.6164) (28.593, 9.6429) (28.7072, 9.6835) knots 0 0 0 0 1 1 1 1
  spline S333 degree 3 poles (28.7072, 9.6835) (28.8285, 9.7266) (28.9387, 9.7894) (29.0323, 9.8713) knots 0 0 0 0 0.99484 0.99484 0.99484 0.99484
  spline S334 degree 3 poles (29.0323, 9.8713) (29.4258, 10.205) (29.6014, 10.7582) (29.6014, 11.4782) knots 0.001205 0.001205 0.001205 0.001205 1 1 1 1
  spline S335 degree 3 poles (29.6014, 11.4782) (29.6014, 11.9835) (29.53, 12.3796) (29.3528, 12.6718) knots 0 0 0 0 1 1 1 1
  spline S336 degree 3 poles (29.3528, 12.6718) (29.1881, 12.9434) (28.9668, 13.138) (28.6989, 13.2204) knots 0.000001 0.000001 0.000001 0.000001 1 1 1 1
  spline S337 degree 3 poles (23.9005, 4.9518) (24.0063, 5.076) (24.0503, 5.2401) (24.0489, 5.4125) knots 0.000001 0.000001 0.000001 0.000001 1 1 1 1
  spline S338 degree 3 poles (24.0489, 5.4125) (24.0478, 5.5555) (24.0078, 5.6948) (23.929, 5.8109) knots 0 0 0 0 1 1 1 1
  spline S339 degree 3 poles (23.929, 5.8109) (23.851, 5.926) (23.7381, 6.0146) (23.6078, 6.0681) knots 0 0 0 0 0.998037 0.998037 0.998037 0.998037
  spline S340 degree 3 poles (23.6078, 6.0681) (23.4494, 6.1336) (23.2625, 6.1401) (22.9793, 6.1379) knots 0 0 0 0 1 1 1 1
  line L130 (22.9793, 6.1379) -> (22.0442, 6.1305)
  line L131 (22.0442, 6.1305) -> (22.056, 4.6494)
  line L132 (22.056, 4.6494) -> (22.9696, 4.6566)
  spline S341 degree 3 poles (22.9696, 4.6566) (23.1725, 4.6582) (23.3484, 4.6766) (23.5012, 4.7166) knots 0 0 0 0 1 1 1 1
  spline S342 degree 3 poles (23.5012, 4.7166) (23.6603, 4.7583) (23.8007, 4.8345) (23.9005, 4.9518) knots 0 0 0 0 1 1 1 1
  line L133 (28.8907, 3.9873) -> (30.6359, 4.0012)
  line L134 (30.6359, 4.0012) -> (29.7362, 6.4048)
  line L135 (29.7362, 6.4048) -> (28.8907, 3.9873)
  circle A4 centre (29.9097, 20.6624) radius 4.2
  dimension "d1" = 60
  dimension "d2" = 35
  dimension "d3" = 5
  dimension "d4" = 11
  dimension "d5" = 1
  dimension "d7" = 6
  dimension "d8" = 8
  dimension "d20" = 0.2
  dimension "d21" = 0.2
  dimension "d22" = 0.2
  dimension "d31" = 0.2
  constraint horizontal L0
  constraint vertical L1
  constraint horizontal L2
  constraint vertical L3
  constraint coincident L0.start L3.end
  constraint vertical L4
  constraint tangent L4 A1
  constraint tangent L5 A1
  constraint vertical L5
  constraint equal L4 L5
  constraint concentric A2 A3
  measures "d1" distance of L0.start L0.end
  measures "d2" distance of L0.start L2.end
  measures "d3" diameter of A0
  measures "d4" diameter of A3
  measures "d5" radius of A1
  measures "d7" distance of L4.start L4.end
  measures "d8" diameter of A2
extrude "Estrusione6" add sketch "Schizzo1" along normal blind 2 contours L0 L1 L2 L3 | L4 L5 A1 A3 | A2 | L6 L7 S0 S1 S2 S3 L8 S4 S5 L9 S6 S7 S8 L10 L11 S9 S10 S11 L12 S12 S13 L13 S14 S15 S16 S17 L14 L15 S18 S19 S20 S21 S22 S23 S24 | L16 S25 S26 S27 S28 L17 S29 S30 S31 S32 | L18 S33 S34 S35 S36 S37 S38 S39 S40 S41 L19 S42 S43 S44 L20 S45 S46 | L21 L22 S47 S48 S49 S50 S51 S52 S53 L23 | L24 L25 L26 S54 S55 S56 S57 L27 L28 S58 S59 S60 S61 L29 S62 S63 S64 L30 S65 S66 S67 S68 | L31 S69 S70 S71 S72 L32 S73 S74 S75 S76 | L33 L34 S77 S78 S79 S80 L35 S81 S82 S83 S84 S85 L36 L37 S86 S87 S88 S89 L38 S90 S91 S92 S93 S94 S95 S96 | L39 L40 L41 S97 S98 S99 S100 L42 L43 L44 S101 S102 S103 S104 L45 S105 S106 L46 S107 S108 S109 L47 S110 S111 S112 S113 | L48 L49 S114 S115 S116 S117 L50 S118 S119 S120 S121 S122 L51 L52 S123 S124 S125 S126 L53 S127 S128 S129 S130 S131 S132 S133 | L54 L55 S134 S135 S136 S137 L56 L57 S138 S139 S140 S141 L58 S142 S143 S144 S145 | L59 L60 L61 S146 S147 S148 S149 L62 L63 L64 S150 S151 S152 S153 L65 S154 S155 L66 S156 S157 S158 L67 S159 S160 S161 S162 | L68 L69 S163 S164 S165 S166 L70 S167 S168 L71 S169 S170 S171 S172 S173 S174 S175 S176 S177 S178 S179 S180 S181 S182 S183 S184 S185 L72 S186 S187 S188 | L73 L74 L75 S189 S190 S191 S192 S193 S194 | L76 L77 S195 S196 S197 S198 L78 L79 S199 S200 S201 S202 L80 S203 S204 S205 S206 | L81 L82 L83 S207 S208 S209 S210 S211 S212 L84 S213 S214 S215 S216 S217 S218 S219 S220 L85 S221 S222 S223 S224 S225 S226 S227 | L86 L87 L88 | L89 S228 S229 S230 S231 L90 S232 S233 S234 S235 | L91 L92 S236 S237 S238 S239 L93 S240 S241 S242 S243 S244 L94 L95 S245 S246 S247 S248 L96 S249 S250 S251 S252 S253 S254 S255 | L97 L98 S256 S257 S258 S259 L99 S260 S261 L100 S262 S263 S264 L101 L102 S265 S266 S267 L103 S268 S269 L104 S270 S271 S272 S273 L105 L106 S274 S275 S276 S277 S278 S279 S280 | L107 L108 L109 S281 S282 S283 S284 L110 L111 L112 S285 S286 S287 S288 L113 S289 S290 L114 S291 S292 S293 L115 S294 S295 S296 S297 | L116 L117 S298 S299 S300 S301 L118 S302 S303 S304 S305 S306 L119 L120 S307 S308 S309 S310 L121 S311 S312 S313 S314 S315 S316 S317 | L122 L123 S318 S319 S320 S321 L124 L125 S322 S323 S324 S325 L126 S326 S327 S328 S329 | S330 L127 L128 L129 S331 S332 S333 S334 S335 S336 | S337 S338 S339 S340 L130 L131 L132 S341 S342 | L133 L134 L135 | A4
extrude "Estrusione7" add sketch "Schizzo1" along normal blind 4 from surface at 2 contours A2
extrude "Estrusione8" add sketch "Schizzo1" along normal blind 4 from surface at 2 contours L21 L22 S47 S48 S49 S50 S51 S52 S53 L23 | L73 L74 L75 S189 S190 S191 S192 S193 S194 | L86 L87 L88
extrude "Estrusione5" [rolled back] along distance 2 taper angle 0
extrude "Estrusione2" [rolled back] along distance 4 taper angle 0
extrude "Estrusione3" [rolled back] along distance 4 taper angle 0
extrude "Estrusione4" [rolled back] along distance 2 taper angle 0
extrude "Estrusione1" [rolled back] along distance 2 taper angle 0
